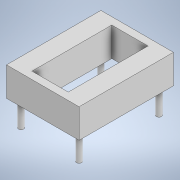
# Autodesk Inventor part: top
Saved by Autodesk Inventor 2022 (Build 260153000, 153)
## iProperties
Created: 2024-03-25
Part Number: top
Material: Generic
Document SubType Name: Modeling
Designer: subin
Density: 1 g/cm^3
Appearance: Default
Author: subin
Autodesk Inventor part; units mm, degrees
ref_plane "YZ Plane" through (0, 0, 0) normal (1, 0, 0) x (0, 1, 0)
ref_plane "XZ Plane" through (0, 0, 0) normal (0, 1, 0) x (-1, 0, 0)
ref_plane "XY Plane" through (0, 0, 0) normal (0, 0, 1) x (1, 0, 0)
sketch "Sketch1" plane through (0, 0, 0) normal (0, 1, 0) x (-1, 0, 0)
  line L0 (0, 0) -> (-100, 0)
  line L1 (-100, 0) -> (-100, -130)
  line L2 (-100, -130) -> (0, -130)
  line L3 (0, -130) -> (0, 0)
  dimension "d0" = 100
  dimension "d1" = 130
  constraints: 8 end point, 2 parallel, 1 horizontal, 1 perpendicular
  measures "d0" distance of L2.end L1.end
  measures "d1" distance of L1.end L0.end
extrude "Extrusion1" add sketch "Sketch1" along normal blind 40
sketch "Sketch2" plane through (0, 40, 0) normal (0, 1, 0) x (1, 0, 0)
  line L0 (25, 10) -> (75, 10)
  line L1 (75, 10) -> (75, 120)
  line L2 (75, 120) -> (25, 120)
  line L3 (25, 120) -> (25, 10)
  line L4 (100, 130) -> (0, 130) projected
  line L5 (0, 0) -> (100, 0) projected
  line L6 (0, 130) -> (0, 0) projected
  line L7 (100, 0) -> (100, 130) projected
  dimension "d4" = 10
  dimension "d5" = 10
  dimension "d6" = 25
  dimension "d7" = 25
  constraints: 8 end point, 2 parallel, 1 horizontal, 1 perpendicular
  measures "d4" distance between parallel lines of L4 L2
  measures "d5" distance between parallel lines of L5 L0
  measures "d6" distance between parallel lines of L6 L3
  measures "d7" distance between parallel lines of L7 L1
extrude "Extrusion2" cut sketch "Sketch2" against normal blind 40 contours L3 L2 L1 L0
sketch "Sketch3" plane through (0, 0, 0) normal (0, -1, 0) x (1, 0, 0)
  circle A0 centre (90, -10) radius 3.5
  line L0 (100, 0) -> (100, -130) projected
  line L1 (0, 0) -> (100, 0) projected
  line L2 (0, 0) -> (100, 0) projected
  line L3 (50, 0) -> (50, -130)
  line L4 (100, 0) -> (100, -130) projected
  line L5 (100, -65) -> (0, -65)
  line L6 (0, -130) -> (0, 0) projected
  circle A1 centre (90, -120) radius 3.5
  circle A2 centre (10, -10) radius 3.5
  line L7 (0, 0) -> (0, -130)
  line L8 (0, 0) -> (0, -130)
  circle A3 centre (10, -120) radius 3.5
  dimension "d10" = 7
  dimension "d11" = 10
  dimension "d12" = 10
  constraints: 8 end point, 4 centre point, 3 midpoint, 3 symmetric about line, 1 vertical, 3 other
  measures "d10" diameter of A0
  measures "d11" distance from line of L0 A0.centre
  measures "d12" distance from line of L1 A0.centre
extrude "Extrusion3" add sketch "Sketch3" along normal blind 35 contours A0 | A1 | A2 | A3
body "Solid1"
